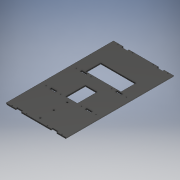
# Autodesk Inventor part: BA11
Saved by Autodesk Inventor 2017 (Build 210142000, 142)
## iProperties
Created: 2019-05-29
Part Number: BA11
Material: Wood (Cherry)
Document SubType Name: Modeling
Designer: Dell
Density: 0.63 g/cm^3
Appearance: Smooth - Black
Mass: 587.672 g
Surface Area: 3107.49 cm^2
Volume: 932.812 cm^3
Author: Dell
Autodesk Inventor part; units mm, degrees
ref_plane "YZ Plane" through (0, 0, 0) normal (1, 0, 0) x (0, 1, 0)
ref_plane "XZ Plane" through (0, 0, 0) normal (0, 1, 0) x (-1, 0, 0)
ref_plane "XY Plane" through (0, 0, 0) normal (0, 0, 1) x (1, 0, 0)
sketch "Sketch1" plane through (0, 0, 0) normal (0, 0, 1) x (1, 0, 0)
  line L0 (0, 0) -> (303.5592, 0)
  line L1 (303.5592, 0) -> (303.5592, 539.75)
  line L2 (303.5592, 539.75) -> (0, 539.75)
  line L3 (0, 539.75) -> (0, 0)
  dimension "d0" = 539.75
  dimension "d1" = 303.5592
  constraints: 8 end point, 2 parallel, 1 horizontal, 1 perpendicular
  measures "d0" distance of L1.end L0.end
  measures "d1" distance of L1.end L2.end
extrude "Extrusion1" add sketch "Sketch1" along normal blind 6.35
sketch "Sketch2" plane through (0, 539.75, 0) normal (0, 1, 0) x (1, 0, 0)
  line L0 (0, -6.35) -> (303.5592, -6.35) projected
  line L1 (0, -6.35) -> (3.6662, 0)
  line L2 (0, 0) -> (303.5592, 0) projected
  line L3 (0, 0) -> (3.6662, 0)
  line L4 (0, 0) -> (0, -6.35)
  line L5 (303.5592, -6.35) -> (299.8931, 0)
  line L6 (303.5592, 0) -> (299.8931, 0)
  line L7 (303.5592, 0) -> (303.5592, -6.35) projected
  line L8 (303.5592, 0) -> (303.5592, -6.35)
  dimension "d4" = 30
  dimension "d5" = 30
  constraints: 12 end point, 2 collinear, 2 point on line, 1 perpendicular, 1 vertical
  measures "d4" angle of L4 L1
  measures "d5" angle of L5 L7
extrude "Extrusion2" cut sketch "Sketch2" against normal through all contours L4 L2 L1 | L5 L2 L7
sketch "Sketch3" plane through (0, 0, 6.35) normal (0, 0, 1) x (1, 0, 0)
  line L0 (50.1796, 532.13) -> (75.5796, 532.13)
  line L1 (75.5796, 532.13) -> (75.5796, 539.75)
  line L2 (75.5796, 539.75) -> (50.1796, 539.75)
  line L3 (50.1796, 539.75) -> (50.1796, 532.13)
  line L4 (303.5592, 539.75) -> (0, 539.75) projected
  line L5 (227.9796, 539.75) -> (253.3796, 539.75)
  line L6 (253.3796, 539.75) -> (253.3796, 532.13)
  line L7 (253.3796, 532.13) -> (227.9796, 532.13)
  line L8 (227.9796, 532.13) -> (227.9796, 539.75)
  line L9 (75.5796, 532.13) -> (227.9796, 532.13) construction
  line L10 (50.1796, 0) -> (75.5796, 0)
  line L11 (75.5796, 0) -> (75.5796, 7.62)
  line L12 (75.5796, 7.62) -> (50.1796, 7.62)
  line L13 (50.1796, 7.62) -> (50.1796, 0)
  line L14 (227.9796, 0) -> (253.3796, 0)
  line L15 (253.3796, 0) -> (253.3796, 7.62)
  line L16 (253.3796, 7.62) -> (227.9796, 7.62)
  line L17 (227.9796, 7.62) -> (227.9796, 0)
  line L18 (0, 0) -> (303.5592, 0) projected
  point P0 (151.7796, 532.13)
  point P1 (151.7796, 539.75)
  dimension "d8" = 7.62
  dimension "d9" = 25.4
  dimension "d10" = 25.4
  dimension "d11" = 152.4
  dimension "d14" = 7.62
  constraints: 34 end point, 8 parallel, 5 horizontal, 5 vertical alignment, 4 perpendicular, 4 point on line, 2 horizontal alignment, 2 midpoint
  measures "d8" distance of L2.end L0.start
  measures "d9" distance of L6.end L7.end
  measures "d10" distance of L0.start L0.end
  measures "d11" distance of L0.end L7.end
  measures "d14" distance of L12.end L10.start
extrude "Extrusion3" cut sketch "Sketch3" against normal through all
sketch "Sketch4" plane through (0, 0, 6.35) normal (0, 0, 1) x (1, 0, 0)
  line L0 (50.1796, 330.2) -> (75.5796, 330.2)
  line L1 (75.5796, 330.2) -> (75.5796, 323.85)
  line L2 (75.5796, 323.85) -> (50.1796, 323.85)
  line L3 (50.1796, 323.85) -> (50.1796, 330.2)
  line L4 (227.9796, 330.2) -> (253.3796, 330.2)
  line L5 (253.3796, 330.2) -> (253.3796, 323.85)
  line L6 (253.3796, 323.85) -> (227.9796, 323.85)
  line L7 (227.9796, 323.85) -> (227.9796, 330.2)
  line L8 (75.5796, 532.13) -> (50.1796, 532.13) projected
  line L9 (253.3796, 532.13) -> (227.9796, 532.13) projected
  line L10 (50.1796, 539.75) -> (0, 539.75) projected
  point P0 (0, 0)
  point P1 (62.8796, 330.2)
  point P2 (62.8796, 532.13)
  point P3 (240.6796, 330.2)
  point P4 (240.6796, 532.13)
  dimension "d15" = 25.4
  dimension "d16" = 6.35
  dimension "d17" = 25.4
  dimension "d18" = 6.35
  dimension "d19" = 209.55
  constraints: 16 end point, 4 midpoint, 4 parallel, 2 horizontal, 2 perpendicular, 2 vertical alignment, 1 horizontal alignment
  measures "d15" distance of L1.end L2.end
  measures "d16" distance of L0.end L1.end
  measures "d17" distance of L5.end L6.end
  measures "d18" distance of L4.end L5.end
  measures "d19" distance between parallel lines of L10 L0
extrude "Extrusion4" cut sketch "Sketch4" against normal through all
sketch "Sketch5" plane through (0, 0, 6.35) normal (0, 0, 1) x (1, 0, 0)
  line L0 (50.1796, 177.8) -> (75.5796, 177.8)
  line L1 (75.5796, 177.8) -> (75.5796, 171.45)
  line L2 (75.5796, 171.45) -> (50.1796, 171.45)
  line L3 (50.1796, 171.45) -> (50.1796, 177.8)
  line L4 (227.9796, 177.8) -> (253.3796, 177.8)
  line L5 (253.3796, 177.8) -> (253.3796, 171.45)
  line L6 (253.3796, 171.45) -> (227.9796, 171.45)
  line L7 (227.9796, 171.45) -> (227.9796, 177.8)
  line L8 (50.1796, 7.62) -> (75.5796, 7.62) projected
  line L9 (227.9796, 7.62) -> (253.3796, 7.62) projected
  line L10 (0, 0) -> (50.1796, 0) projected
  point P0 (62.8796, 171.45)
  point P1 (62.8796, 7.62)
  point P2 (240.6796, 171.45)
  point P3 (240.6796, 7.62)
  dimension "d22" = 25.4
  dimension "d23" = 6.35
  dimension "d24" = 25.4
  dimension "d25" = 6.35
  dimension "d26" = 177.8
  constraints: 16 end point, 4 midpoint, 4 parallel, 2 horizontal, 2 perpendicular, 2 vertical alignment, 1 horizontal alignment
  measures "d22" distance of L1.end L2.end
  measures "d23" distance of L0.end L1.end
  measures "d24" distance of L5.end L6.end
  measures "d25" distance of L4.end L5.end
  measures "d26" distance between parallel lines of L10 L0
extrude "Extrusion5" cut sketch "Sketch5" against normal through all
sketch "Sketch6" plane through (0, 0, 6.35) normal (0, 0, 1) x (1, 0, 0)
  line L0 (240.6796, 336.55) -> (62.8796, 336.55)
  line L1 (62.8796, 336.55) -> (62.8796, 412.75)
  line L2 (62.8796, 412.75) -> (240.6796, 412.75)
  line L3 (240.6796, 412.75) -> (240.6796, 336.55)
  line L4 (75.5796, 0) -> (227.9796, 0) projected
  line L5 (227.9796, 539.75) -> (75.5796, 539.75) projected
  point P0 (0, 0)
  point P1 (151.7796, 336.55)
  point P2 (151.7796, 0)
  dimension "d29" = 177.8
  dimension "d30" = 76.2
  dimension "d31" = 127
  constraints: 8 end point, 2 midpoint, 2 parallel, 1 horizontal, 1 perpendicular, 1 vertical alignment
  measures "d29" distance of L0.start L0.end
  measures "d30" distance of L0.end L1.end
  measures "d31" distance between parallel lines of L5 L2
extrude "Extrusion6" cut sketch "Sketch6" against normal through all
sketch "Sketch7" plane through (0, 0, 6.35) normal (0, 0, 1) x (1, 0, 0)
  line L0 (181.7796, 176.55) -> (121.7796, 176.55)
  line L1 (121.7796, 176.55) -> (121.7796, 276.55)
  line L2 (121.7796, 276.55) -> (181.7796, 276.55)
  line L3 (181.7796, 276.55) -> (181.7796, 176.55)
  line L4 (240.6796, 336.55) -> (62.8796, 336.55) projected
  point P0 (0, 0)
  point P1 (151.7796, 336.55)
  point P2 (151.7796, 276.55)
  dimension "d34" = 60
  dimension "d35" = 100
  dimension "d36" = 60
  constraints: 8 end point, 2 midpoint, 2 parallel, 1 horizontal, 1 perpendicular, 1 vertical alignment
  measures "d34" distance of L1.end L2.end
  measures "d35" distance of L0.end L1.end
  measures "d36" distance between parallel lines of L4 L2
extrude "Extrusion7" cut sketch "Sketch7" against normal through all
sketch "Sketch8" plane through (0, 0, 6.35) normal (0, 0, 1) x (1, 0, 0)
  circle A0 centre (26.2013, 535.94) radius 2.25
  circle A1 centre (99.558, 535.94) radius 2.25
  circle A2 centre (204.0013, 535.94) radius 2.25
  circle A3 centre (277.358, 535.94) radius 2.25
  line L0 (50.1796, 532.13) -> (50.1796, 539.75) projected
  line L1 (26.2013, 535.94) -> (99.558, 535.94) construction
  line L2 (204.0013, 535.94) -> (277.358, 535.94) construction
  line L3 (253.3796, 532.13) -> (227.9796, 532.13) projected
  line L4 (75.5796, 532.13) -> (50.1796, 532.13) projected
  circle A4 centre (26.2013, 327.025) radius 2.25
  circle A5 centre (99.558, 327.025) radius 2.25
  circle A6 centre (204.0013, 327.025) radius 2.25
  circle A7 centre (277.358, 327.025) radius 2.25
  line L5 (50.1796, 323.85) -> (50.1796, 330.2) projected
  circle A8 centre (26.2013, 174.625) radius 2.25
  circle A9 centre (99.558, 174.625) radius 2.25
  circle A10 centre (204.0013, 174.625) radius 2.25
  circle A11 centre (277.358, 174.625) radius 2.25
  circle A12 centre (277.358, 3.81) radius 2.25
  circle A13 centre (204.0013, 3.81) radius 2.25
  circle A14 centre (99.558, 3.81) radius 2.25
  circle A15 centre (26.2013, 3.81) radius 2.25
  line L6 (50.1796, 171.45) -> (50.1796, 177.8) projected
  line L7 (50.1796, 0) -> (50.1796, 7.62) projected
  point P0 (0, 0)
  point P1 (50.1796, 535.94)
  point P2 (50.1796, 535.94)
  point P3 (240.6796, 535.94)
  point P4 (240.6796, 532.13)
  point P5 (62.8796, 535.94)
  point P6 (62.8796, 532.13)
  point P7 (50.1796, 327.025)
  point P8 (50.1796, 174.625)
  point P9 (50.1796, 3.81)
  dimension "d39" = 4.5
  dimension "d40" = 4.5
  dimension "d41" = 4.5
  dimension "d42" = 4.5
  dimension "d43" = 73.3567
  dimension "d44" = 73.3567
  dimension "d45" = 4.5
  dimension "d46" = 4.5
  dimension "d47" = 4.5
  dimension "d48" = 4.5
  dimension "d49" = 4.5
  dimension "d50" = 4.5
  dimension "d51" = 4.5
  dimension "d52" = 4.5
  dimension "d53" = 4.5
  dimension "d54" = 4.5
  dimension "d55" = 4.5
  dimension "d56" = 4.5
  constraints: 16 centre point, 16 horizontal alignment, 14 vertical alignment, 9 midpoint, 4 end point, 2 horizontal
  measures "d39" diameter of A0
  measures "d40" diameter of A1
  measures "d41" diameter of A2
  measures "d42" diameter of A3
  measures "d43" distance of L1.start L1.end
  measures "d44" distance of L2.start L2.end
  measures "d45" diameter of A4
  measures "d46" diameter of A5
  measures "d47" diameter of A6
  measures "d48" diameter of A7
  measures "d49" diameter of A8
  measures "d50" diameter of A9
  measures "d51" diameter of A10
  measures "d52" diameter of A11
  measures "d53" diameter of A12
  measures "d54" diameter of A13
  measures "d55" diameter of A14
  measures "d56" diameter of A15
extrude "Extrusion8" cut sketch "Sketch8" against normal through all
sketch "Sketch9" plane through (0, 0, 6.35) normal (0, 0, 1) x (1, 0, 0)
  circle A0 centre (151.7796, 155.42) radius 4
  circle A1 centre (151.7796, 87.71) radius 4
  circle A2 centre (151.7796, 20) radius 4
  line L0 (75.5796, 0) -> (227.9796, 0) projected
  point P0 (0, 0)
  point P1 (151.7796, 0)
  dimension "d59" = 20
  dimension "d60" = 8
  dimension "d61" = 8
  dimension "d62" = 8
  dimension "d63" = 67.71
  dimension "d64" = 67.71
  constraints: 3 centre point, 3 vertical alignment, 1 midpoint
  measures "d59" distance from line of L0 A2.centre
  measures "d60" diameter of A2
  measures "d61" diameter of A1
  measures "d62" diameter of A0
  measures "d63" distance of A2.centre A1.centre
  measures "d64" distance of A0.centre A1.centre
extrude "Extrusion9" cut sketch "Sketch9" against normal through all
sketch "Sketch10" plane through (0, 0, 6.35) normal (0, 0, 1) x (1, 0, 0)
  circle A0 centre (151.7796, 87.71) radius 4 construction
  circle A1 centre (151.7796, 155.42) radius 4 construction
  circle A2 centre (151.7796, 20) radius 4 construction
  circle A3 centre (99.558, 3.81) radius 2.25 construction
  circle A4 centre (277.358, 3.81) radius 2.25 construction
  circle A5 centre (204.0013, 174.625) radius 2.25 construction
  circle A6 centre (26.2013, 174.625) radius 2.25 construction
  circle A7 centre (204.0013, 327.025) radius 2.25 construction
  circle A8 centre (26.2013, 327.025) radius 2.25 construction
  circle A9 centre (204.0013, 535.94) radius 2.25 construction
  circle A10 centre (26.2013, 535.94) radius 2.25 construction
  circle A11 centre (99.558, 535.94) radius 2.25 construction
  circle A12 centre (277.358, 535.94) radius 2.25 construction
  circle A13 centre (99.558, 327.025) radius 2.25 construction
  circle A14 centre (277.358, 327.025) radius 2.25 construction
  circle A15 centre (99.558, 174.625) radius 2.25 construction
  circle A16 centre (277.358, 174.625) radius 2.25 construction
  circle A17 centre (204.0013, 3.81) radius 2.25 construction
  circle A18 centre (26.2013, 3.81) radius 2.25 construction
  line L0 (181.7796, 276.55) -> (181.7796, 176.55) construction
  line L1 (181.7796, 176.55) -> (121.7796, 176.55) construction
  line L2 (121.7796, 176.55) -> (121.7796, 276.55) construction
  line L3 (121.7796, 276.55) -> (181.7796, 276.55) construction
  line L4 (240.6796, 412.75) -> (240.6796, 336.55) construction
  line L5 (240.6796, 336.55) -> (62.8796, 336.55) construction
  line L6 (62.8796, 336.55) -> (62.8796, 412.75) construction
  line L7 (62.8796, 412.75) -> (240.6796, 412.75) construction
  line L8 (50.1796, 171.45) -> (50.1796, 177.8) construction
  line L9 (50.1796, 177.8) -> (75.5796, 177.8) construction
  line L10 (75.5796, 177.8) -> (75.5796, 171.45) construction
  line L11 (75.5796, 171.45) -> (50.1796, 171.45) construction
  line L12 (227.9796, 171.45) -> (227.9796, 177.8) construction
  line L13 (227.9796, 177.8) -> (253.3796, 177.8) construction
  line L14 (253.3796, 177.8) -> (253.3796, 171.45) construction
  line L15 (253.3796, 171.45) -> (227.9796, 171.45) construction
  line L16 (50.1796, 323.85) -> (50.1796, 330.2) construction
  line L17 (50.1796, 330.2) -> (75.5796, 330.2) construction
  line L18 (75.5796, 330.2) -> (75.5796, 323.85) construction
  line L19 (75.5796, 323.85) -> (50.1796, 323.85) construction
  line L20 (227.9796, 323.85) -> (227.9796, 330.2) construction
  line L21 (227.9796, 330.2) -> (253.3796, 330.2) construction
  line L22 (253.3796, 330.2) -> (253.3796, 323.85) construction
  line L23 (253.3796, 323.85) -> (227.9796, 323.85) construction
  line L24 (50.1796, 0) -> (50.1796, 7.62) construction
  line L25 (50.1796, 7.62) -> (75.5796, 7.62) construction
  line L26 (75.5796, 7.62) -> (75.5796, 0) construction
  line L27 (75.5796, 0) -> (227.9796, 0) construction
  line L28 (227.9796, 0) -> (227.9796, 7.62) construction
  line L29 (227.9796, 7.62) -> (253.3796, 7.62) construction
  line L30 (253.3796, 7.62) -> (253.3796, 0) construction
  line L31 (253.3796, 0) -> (303.5592, 0) construction
  line L32 (303.5592, 0) -> (303.5592, 539.75) construction
  line L33 (303.5592, 539.75) -> (253.3796, 539.75) construction
  line L34 (253.3796, 539.75) -> (253.3796, 532.13) construction
  line L35 (253.3796, 532.13) -> (227.9796, 532.13) construction
  line L36 (227.9796, 532.13) -> (227.9796, 539.75) construction
  line L37 (227.9796, 539.75) -> (75.5796, 539.75) construction
  line L38 (75.5796, 539.75) -> (75.5796, 532.13) construction
  line L39 (75.5796, 532.13) -> (50.1796, 532.13) construction
  line L40 (50.1796, 532.13) -> (50.1796, 539.75) construction
  line L41 (50.1796, 539.75) -> (0, 539.75) construction
  line L42 (0, 539.75) -> (0, 0) construction
  line L43 (0, 0) -> (50.1796, 0) construction
  line L44 (48.9096, 539.75) -> (76.8496, 539.75)
  line L45 (76.8496, 539.75) -> (76.8496, 532.13)
  line L46 (76.8496, 532.13) -> (48.9096, 532.13)
  line L47 (48.9096, 532.13) -> (48.9096, 539.75)
  line L48 (226.7096, 539.75) -> (254.6496, 539.75)
  line L49 (254.6496, 539.75) -> (254.6496, 532.13)
  line L50 (254.6496, 532.13) -> (226.7096, 532.13)
  line L51 (226.7096, 532.13) -> (226.7096, 539.75)
  line L52 (48.9096, 331.47) -> (76.8496, 331.47)
  line L53 (76.8496, 331.47) -> (76.8496, 322.58)
  line L54 (76.8496, 322.58) -> (48.9096, 322.58)
  line L55 (48.9096, 322.58) -> (48.9096, 331.47)
  line L56 (226.7096, 331.47) -> (254.6496, 331.47)
  line L57 (254.6496, 331.47) -> (254.6496, 322.58)
  line L58 (254.6496, 322.58) -> (226.7096, 322.58)
  line L59 (226.7096, 322.58) -> (226.7096, 331.47)
  line L60 (48.9096, 179.07) -> (76.8496, 179.07)
  line L61 (76.8496, 179.07) -> (76.8496, 170.18)
  line L62 (76.8496, 170.18) -> (48.9096, 170.18)
  line L63 (48.9096, 170.18) -> (48.9096, 179.07)
  line L64 (226.7096, 179.07) -> (254.6496, 179.07)
  line L65 (254.6496, 179.07) -> (254.6496, 170.18)
  line L66 (254.6496, 170.18) -> (226.7096, 170.18)
  line L67 (226.7096, 170.18) -> (226.7096, 179.07)
  line L68 (3.6662, 0) -> (50.1796, 0) projected
  line L69 (48.9096, 0) -> (76.8496, 0)
  line L70 (76.8496, 0) -> (76.8496, 7.62)
  line L71 (76.8496, 7.62) -> (48.9096, 7.62)
  line L72 (48.9096, 7.62) -> (48.9096, 0)
  line L73 (75.5796, 0) -> (227.9796, 0) projected
  line L74 (226.7096, 0) -> (254.6496, 0)
  line L75 (254.6496, 0) -> (254.6496, 7.62)
  line L76 (254.6496, 7.62) -> (226.7096, 7.62)
  line L77 (226.7096, 7.62) -> (226.7096, 0)
  line L78 (253.3796, 532.13) -> (227.9796, 532.13) projected
  line L79 (227.9796, 7.62) -> (253.3796, 7.62) projected
  point P0 (62.8796, 532.13)
  point P1 (240.6796, 532.13)
  point P2 (240.6796, 532.13)
  point P3 (62.8796, 7.62)
  point P4 (240.6796, 7.62)
  point P5 (240.6796, 7.62)
  point P6 (50.1796, 327.025)
  point P7 (48.9096, 327.025)
  point P8 (227.9796, 327.025)
  point P9 (226.7096, 327.025)
  point P10 (227.9796, 174.625)
  point P11 (226.7096, 174.625)
  point P12 (50.1796, 174.625)
  point P13 (48.9096, 174.625)
  point P14 (62.8796, 330.2)
  point P15 (62.8796, 331.47)
  point P16 (240.6796, 330.2)
  point P17 (240.6796, 331.47)
  point P18 (240.6796, 177.8)
  point P19 (240.6796, 179.07)
  point P20 (62.8796, 177.8)
  point P21 (62.8796, 179.07)
  dimension "d67" = 1.27
  dimension "d68" = 1.27
  dimension "d69" = 1.27
  dimension "d70" = 1.27
  dimension "d71" = 1.27
  dimension "d72" = 1.27
  dimension "d73" = 1.27
  dimension "d74" = 1.27
  dimension "d75" = 1.27
  dimension "d76" = 1.27
  dimension "d77" = 1.27
  constraints: 64 end point, 28 midpoint, 16 parallel, 8 horizontal, 8 perpendicular, 7 point on line, 4 horizontal alignment, 4 vertical alignment
  measures "d67" distance between parallel lines of L51 L36
  measures "d68" distance between parallel lines of L40 L47
  measures "d69" distance between parallel lines of L24 L72
  measures "d70" distance between parallel lines of L77 L28
  measures "d71" distance between parallel lines of L52 L17
  measures "d72" distance between parallel lines of L16 L55
  measures "d73" distance between parallel lines of L56 L21
  measures "d74" distance between parallel lines of L64 L13
  measures "d75" distance between parallel lines of L12 L67
  measures "d76" distance between parallel lines of L61 L10
  measures "d77" distance between parallel lines of L60 L9
extrude "Extrusion10" cut sketch "Sketch10" against normal through all
sketch "Sketch11" plane through (0, 0, 6.35) normal (0, 0, 1) x (1, 0, 0)
  line L0 (76.8496, 7.62) -> (76.8496, 0) construction
  line L1 (76.8496, 0) -> (226.7096, 0) construction
  line L2 (226.7096, 0) -> (226.7096, 7.62) construction
  line L3 (226.7096, 7.62) -> (254.6496, 7.62) construction
  line L4 (254.6496, 7.62) -> (254.6496, 0) construction
  line L5 (254.6496, 0) -> (303.5592, 0) construction
  line L6 (303.5592, 0) -> (303.5592, 539.75) construction
  line L7 (303.5592, 539.75) -> (254.6496, 539.75) construction
  line L8 (254.6496, 539.75) -> (254.6496, 532.13) construction
  line L9 (254.6496, 532.13) -> (226.7096, 532.13) construction
  line L10 (226.7096, 532.13) -> (226.7096, 539.75) construction
  line L11 (226.7096, 539.75) -> (76.8496, 539.75) construction
  line L12 (76.8496, 539.75) -> (76.8496, 532.13) construction
  line L13 (76.8496, 532.13) -> (48.9096, 532.13) construction
  line L14 (48.9096, 532.13) -> (48.9096, 539.75) construction
  line L15 (48.9096, 539.75) -> (0, 539.75) construction
  line L16 (0, 539.75) -> (0, 0) construction
  line L17 (0, 0) -> (48.9096, 0) construction
  line L18 (48.9096, 0) -> (48.9096, 7.62) construction
  line L19 (48.9096, 7.62) -> (76.8496, 7.62) construction
  line L20 (48.9096, 170.18) -> (48.9096, 179.07) construction
  line L21 (48.9096, 179.07) -> (76.8496, 179.07) construction
  line L22 (76.8496, 179.07) -> (76.8496, 170.18) construction
  line L23 (76.8496, 170.18) -> (48.9096, 170.18) construction
  line L24 (48.9096, 322.58) -> (48.9096, 331.47) construction
  line L25 (48.9096, 331.47) -> (76.8496, 331.47) construction
  line L26 (76.8496, 331.47) -> (76.8496, 322.58) construction
  line L27 (76.8496, 322.58) -> (48.9096, 322.58) construction
  line L28 (226.7096, 322.58) -> (226.7096, 331.47) construction
  line L29 (226.7096, 331.47) -> (254.6496, 331.47) construction
  line L30 (254.6496, 331.47) -> (254.6496, 322.58) construction
  line L31 (254.6496, 322.58) -> (226.7096, 322.58) construction
  line L32 (226.7096, 170.18) -> (226.7096, 179.07) construction
  line L33 (226.7096, 179.07) -> (254.6496, 179.07) construction
  line L34 (254.6496, 179.07) -> (254.6496, 170.18) construction
  line L35 (254.6496, 170.18) -> (226.7096, 170.18) construction
  circle A0 centre (151.7796, 87.71) radius 4 construction
  circle A1 centre (151.7796, 155.42) radius 4 construction
  circle A2 centre (151.7796, 20) radius 4 construction
  circle A3 centre (99.558, 3.81) radius 2.25 construction
  circle A4 centre (277.358, 3.81) radius 2.25 construction
  circle A5 centre (204.0013, 174.625) radius 2.25 construction
  circle A6 centre (26.2013, 174.625) radius 2.25 construction
  circle A7 centre (204.0013, 327.025) radius 2.25 construction
  circle A8 centre (26.2013, 327.025) radius 2.25 construction
  circle A9 centre (204.0013, 535.94) radius 2.25 construction
  circle A10 centre (26.2013, 535.94) radius 2.25 construction
  circle A11 centre (99.558, 535.94) radius 2.25 construction
  circle A12 centre (277.358, 535.94) radius 2.25 construction
  circle A13 centre (99.558, 327.025) radius 2.25 construction
  circle A14 centre (277.358, 327.025) radius 2.25 construction
  circle A15 centre (99.558, 174.625) radius 2.25 construction
  circle A16 centre (277.358, 174.625) radius 2.25 construction
  circle A17 centre (204.0013, 3.81) radius 2.25 construction
  circle A18 centre (26.2013, 3.81) radius 2.25 construction
  line L36 (181.7796, 276.55) -> (181.7796, 176.55) construction
  line L37 (181.7796, 176.55) -> (121.7796, 176.55) construction
  line L38 (121.7796, 176.55) -> (121.7796, 276.55) construction
  line L39 (121.7796, 276.55) -> (181.7796, 276.55) construction
  line L40 (240.6796, 412.75) -> (240.6796, 336.55) construction
  line L41 (240.6796, 336.55) -> (62.8796, 336.55) construction
  line L42 (62.8796, 336.55) -> (62.8796, 412.75) construction
  line L43 (62.8796, 412.75) -> (240.6796, 412.75) construction
  line L44 (-2.2451, -2.2451) -> (-2.2451, 541.9951) construction
  line L45 (-2.2451, 541.9951) -> (51.1547, 541.9951) construction
  line L46 (51.1547, 541.9951) -> (51.1547, 534.3751) construction
  line L47 (51.1547, 534.3751) -> (74.6045, 534.3751) construction
  line L48 (74.6045, 534.3751) -> (74.6045, 541.9951) construction
  line L49 (74.6045, 541.9951) -> (228.9547, 541.9951) construction
  line L50 (228.9547, 541.9951) -> (228.9547, 534.3751) construction
  line L51 (228.9547, 534.3751) -> (252.4045, 534.3751) construction
  line L52 (252.4045, 534.3751) -> (252.4045, 541.9951) construction
  line L53 (252.4045, 541.9951) -> (305.8043, 541.9951) construction
  line L54 (305.8043, 541.9951) -> (305.8043, -2.2451) construction
  line L55 (305.8043, -2.2451) -> (252.4045, -2.2451) construction
  line L56 (252.4045, -2.2451) -> (252.4045, 5.3749) construction
  line L57 (252.4045, 5.3749) -> (228.9547, 5.3749) construction
  line L58 (228.9547, 5.3749) -> (228.9547, -2.2451) construction
  line L59 (228.9547, -2.2451) -> (74.6045, -2.2451) construction
  line L60 (74.6045, -2.2451) -> (74.6045, 5.3749) construction
  line L61 (74.6045, 5.3749) -> (51.1547, 5.3749) construction
  line L62 (51.1547, 5.3749) -> (51.1547, -2.2451) construction
  line L63 (51.1547, -2.2451) -> (-2.2451, -2.2451) construction
  line L64 (74.6045, 329.2249) -> (51.1547, 329.2249) construction
  line L65 (51.1547, 329.2249) -> (51.1547, 324.8251) construction
  line L66 (51.1547, 324.8251) -> (74.6045, 324.8251) construction
  line L67 (74.6045, 324.8251) -> (74.6045, 329.2249) construction
  line L68 (74.6045, 176.8249) -> (51.1547, 176.8249) construction
  line L69 (51.1547, 176.8249) -> (51.1547, 172.4251) construction
  line L70 (51.1547, 172.4251) -> (74.6045, 172.4251) construction
  line L71 (74.6045, 172.4251) -> (74.6045, 176.8249) construction
  line L72 (252.4045, 176.8249) -> (228.9547, 176.8249) construction
  line L73 (228.9547, 176.8249) -> (228.9547, 172.4251) construction
  line L74 (228.9547, 172.4251) -> (252.4045, 172.4251) construction
  line L75 (252.4045, 172.4251) -> (252.4045, 176.8249) construction
  line L76 (252.4045, 329.2249) -> (228.9547, 329.2249) construction
  line L77 (228.9547, 329.2249) -> (228.9547, 324.8251) construction
  line L78 (228.9547, 324.8251) -> (252.4045, 324.8251) construction
  line L79 (252.4045, 324.8251) -> (252.4045, 329.2249) construction
  circle A19 centre (51.1547, 534.3751) radius 3.175
  circle A20 centre (74.6045, 534.3751) radius 3.175
  circle A21 centre (228.9547, 534.3751) radius 3.175
  circle A22 centre (252.4045, 534.3751) radius 3.175
  circle A23 centre (252.4045, 329.2249) radius 3.175
  circle A24 centre (228.9547, 329.2249) radius 3.175
  circle A25 centre (228.9547, 324.8251) radius 3.175
  circle A26 centre (252.4045, 324.8251) radius 3.175
  circle A27 centre (74.6045, 329.2249) radius 3.175
  line L80 (76.8496, 331.47) -> (76.8496, 322.58) projected
  circle A28 centre (74.6045, 324.8251) radius 3.175
  line L81 (48.9096, 322.58) -> (48.9096, 331.47) projected
  circle A29 centre (51.1547, 324.8251) radius 3.175
  circle A30 centre (51.1547, 329.2249) radius 3.175
  circle A31 centre (51.1547, 176.8249) radius 3.175
  circle A32 centre (51.1547, 172.4251) radius 3.175
  circle A33 centre (74.6045, 176.8249) radius 3.175
  line L82 (76.8496, 179.07) -> (76.8496, 170.18) projected
  circle A34 centre (74.6045, 172.4251) radius 3.175
  line L83 (226.7096, 179.07) -> (254.6496, 179.07) projected
  circle A35 centre (228.9547, 176.8249) radius 3.175
  circle A36 centre (228.9547, 172.4251) radius 3.175
  circle A37 centre (252.4045, 172.4251) radius 3.175
  circle A38 centre (252.4045, 176.8249) radius 3.175
  circle A39 centre (252.4045, 5.3749) radius 3.175
  line L84 (226.7096, 0) -> (226.7096, 7.62) projected
  circle A40 centre (228.9547, 5.3749) radius 3.175
  circle A41 centre (74.6045, 5.3749) radius 3.175
  line L85 (48.9096, 7.62) -> (76.8496, 7.62) projected
  circle A42 centre (51.1547, 5.3749) radius 3.175
  dimension "d80" = 6.35
  dimension "d81" = 6.35
  dimension "d82" = 6.35
  dimension "d83" = 6.35
  dimension "d84" = 6.35
  constraints: 72 end point, 24 coincident, 103 other
extrude "Extrusion11" cut sketch "Sketch11" against normal through all
equation "\"d2\" = Panel_Thickness"
equation "\"d8\" = Panel_Thickness + Fit_Tolerance"
equation "\"d14\" = Panel_Thickness + Fit_Tolerance"
equation "\"d16\" = Panel_Thickness"
equation "\"d18\" = Panel_Thickness"
equation "\"d23\" = Panel_Thickness"
equation "\"d25\" = Panel_Thickness"
equation "\"d67\" = Fit_Tolerance"
equation "\"d68\" = Fit_Tolerance"
equation "\"d69\" = Fit_Tolerance"
equation "\"d70\" = Fit_Tolerance"
equation "\"d71\" = Fit_Tolerance"
equation "\"d72\" = Fit_Tolerance"
equation "\"d73\" = Fit_Tolerance"
equation "\"d74\" = Fit_Tolerance"
equation "\"d75\" = Fit_Tolerance"
equation "\"d76\" = Fit_Tolerance"
equation "\"d77\" = Fit_Tolerance"
equation "\"d80\" = Tool_Dia"
equation "\"d81\" = Tool_Dia"
equation "\"d82\" = Tool_Dia"
equation "\"d83\" = Tool_Dia"
equation "\"d84\" = Tool_Dia"
equation "\"Panel_Thickness\" = 6.35"
equation "\"Fit_Tolerance\" = 1.27"
equation "\"Tool_Dia\" = 6.35"
body "Solid1"
